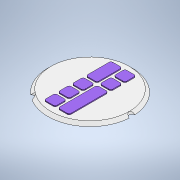
# Autodesk Inventor part: Лого ШП
Saved by Autodesk Inventor 2020 (Build 240168000, 168)
## iProperties
Created: 2021-06-18
Part Number: Лого ШП
Material: Типовые
Document SubType Name: Modeling
Designer: Антон
Density: 1 g/cm^3
Appearance: Белый
Author: Антон
Autodesk Inventor part; units mm, degrees
ref_plane "YZ Plane" through (0, 0, 0) normal (1, 0, 0) x (0, 1, 0)
ref_plane "XZ Plane" through (0, 0, 0) normal (0, 1, 0) x (-1, 0, 0)
ref_plane "XY Plane" through (0, 0, 0) normal (0, 0, 1) x (1, 0, 0)
sketch "Эскиз1" plane through (0, 0, 0) normal (0, 1, 0) x (-1, 0, 0)
  line L0 (0, 0) -> (23.1579, 0)
  line L1 (23.1579, 0) -> (23.1579, -40)
  line L2 (23.1579, -40) -> (0, -40)
  line L3 (0, -40) -> (0, 0)
  line L4 (17.9579, -3) -> (12.2807, -3)
  line L5 (12.2807, -3) -> (12.2807, -8.6772)
  line L6 (12.2807, -8.6772) -> (17.9579, -8.6772)
  line L7 (17.9579, -8.6772) -> (17.9579, -3)
  line L8 (17.9579, -10.0807) -> (12.2807, -10.0807)
  line L9 (12.2807, -10.0807) -> (12.2807, -15.7579)
  line L10 (12.2807, -15.7579) -> (17.9579, -15.7579)
  line L11 (17.9579, -15.7579) -> (17.9579, -10.0807)
  line L12 (17.9579, -17.1614) -> (12.2807, -17.1614)
  line L13 (12.2807, -17.1614) -> (12.2807, -22.8386)
  line L14 (12.2807, -22.8386) -> (17.9579, -22.8386)
  line L15 (17.9579, -22.8386) -> (17.9579, -17.1614)
  line L16 (17.9579, -24.2421) -> (12.2807, -24.2421)
  line L17 (12.2807, -24.2421) -> (12.2807, -37)
  line L18 (12.2807, -37) -> (17.9579, -37)
  line L19 (17.9579, -37) -> (17.9579, -24.2421)
  line L20 (10.8772, -24.2421) -> (5.2, -24.2421)
  line L21 (5.2, -24.2421) -> (5.2, -29.9193)
  line L22 (5.2, -29.9193) -> (10.8772, -29.9193)
  line L23 (10.8772, -29.9193) -> (10.8772, -24.2421)
  line L24 (10.8772, -31.3228) -> (5.2, -31.3228)
  line L25 (5.2, -31.3228) -> (5.2, -37)
  line L26 (5.2, -37) -> (10.8772, -37)
  line L27 (10.8772, -37) -> (10.8772, -31.3228)
  line L28 (10.8772, -3) -> (5.2, -3)
  line L29 (5.2, -3) -> (5.2, -22.8386)
  line L30 (5.2, -22.8386) -> (10.8772, -22.8386)
  line L31 (10.8772, -22.8386) -> (10.8772, -3)
  line L32 (15.1193, -8.6772) -> (15.1193, -10.0807)
  line L33 (15.1193, -15.7579) -> (15.1193, -17.1614)
  line L34 (15.1193, -22.8386) -> (15.1193, -24.2421)
  line L35 (8.0386, -22.8386) -> (8.0386, -24.2421)
  line L36 (8.0386, -29.9193) -> (8.0386, -31.3228)
  line L37 (15.1193, -3) -> (15.1193, 0)
  line L38 (15.1193, -37) -> (15.1193, -40)
  line L39 (17.9579, -12.9193) -> (23.1579, -12.9193)
  line L40 (5.2, -12.9193) -> (0, -12.9193)
  line L41 (12.2807, -12.9193) -> (10.8772, -12.9193)
  dimension "d0" = 23.1579
  dimension "d1" = 40
  dimension "d9" = 5.2
  dimension "d21" = 3
  constraints: 84 end point, 17 equal length, 16 midpoint, 16 parallel, 11 perpendicular, 9 collinear, 8 horizontal, 4 point on line, 1 vertical
  measures "d0" distance of L1.end L2.end
  measures "d1" distance of L0.end L1.end
  measures "d9" distance of L39.start L39.end
  measures "d21" distance of L37.start L37.end
extrude "Выдавливание1" add sketch "Эскиз1" along normal blind 0.5 contours L24 L27 L26 L25 | L20 L23 L22 L21 | L4 L7 L6 L5 | L29 L28 L31 L30 | L11 L10 L9 L8 | L18 L17 L16 L19 | L12 L15 L14 L13
sketch "Эскиз2" plane through (0, 0, 0) normal (0, -1, 0) x (1, 0, 0)
  line L0 (-5.2, -22.8386) -> (-10.8772, -22.8386) projected
  line L1 (-10.8772, -22.8386) -> (-10.8772, -3) projected
  line L2 (-10.8772, -3) -> (-5.2, -3) projected
  line L3 (-5.2, -3) -> (-5.2, -22.8386) projected
  line L4 (-5.2, -31.3228) -> (-5.2, -37) projected
  line L5 (-5.2, -37) -> (-10.8772, -37) projected
  line L6 (-10.8772, -37) -> (-10.8772, -31.3228) projected
  line L7 (-10.8772, -31.3228) -> (-5.2, -31.3228) projected
  line L8 (-17.9579, -17.1614) -> (-12.2807, -17.1614) projected
  line L9 (-12.2807, -22.8386) -> (-17.9579, -22.8386) projected
  line L10 (-17.9579, -22.8386) -> (-17.9579, -17.1614) projected
  line L11 (-17.9579, -37) -> (-17.9579, -24.2421) projected
  line L12 (-17.9579, -24.2421) -> (-12.2807, -24.2421) projected
  line L13 (-12.2807, -37) -> (-17.9579, -37) projected
  line L14 (-12.2807, -15.7579) -> (-17.9579, -15.7579) projected
  line L15 (-17.9579, -15.7579) -> (-17.9579, -10.0807) projected
  line L16 (-17.9579, -10.0807) -> (-12.2807, -10.0807) projected
  line L17 (-17.9579, -8.6772) -> (-17.9579, -3) projected
  line L18 (-17.9579, -3) -> (-12.2807, -3) projected
  line L19 (-12.2807, -8.6772) -> (-17.9579, -8.6772) projected
  line L20 (-5.2, -24.2421) -> (-5.2, -29.9193) projected
  line L21 (-5.2, -29.9193) -> (-10.8772, -29.9193) projected
  line L22 (-10.8772, -29.9193) -> (-10.8772, -24.2421) projected
  line L23 (-10.8772, -24.2421) -> (-5.2, -24.2421) projected
  line L24 (-12.2807, -17.1614) -> (-12.2807, -22.8386) projected
  line L25 (-12.2807, -24.2421) -> (-12.2807, -37) projected
  line L26 (-12.2807, -10.0807) -> (-12.2807, -15.7579) projected
  line L27 (-12.2807, -3) -> (-12.2807, -8.6772) projected
  line L28 (-10.8772, -3) -> (-5.2, -3) projected
  line L29 (-17.9579, -37) -> (-5.2, -3)
  circle A0 centre (-11.5789, -20) radius 21.35
  dimension "d24" = 42.7
  constraints: 2 end point, 1 centre point, 1 midpoint
  measures "d24" diameter of A0
extrude "Выдавливание2" add sketch "Эскиз2" along normal blind 1.5 contours L12 L25 L13 L29 | L29 L11 L12 | L24 L9 L29 | L29 L9 L10 L8 L24 | L0 L1 L29 L3 | L29 L1 L2 | L4 L5 L6 L7 | L14 L15 L16 L26 | L17 L18 L27 L19 | L20 L21 L22 L23 | A0
fillet "Сопряжение1" radius 1 28 edges at (-17.9579, 0.25, -3) (-17.9579, 0.25, -8.6772) (-12.2807, 0.25, -3) (-12.2807, 0.25, -8.6772) (-17.9579, 0.25, -15.7579) (-17.9579, 0.25, -10.0807) (-12.2807, 0.25, -10.0807) (-12.2807, 0.25, -15.7579) (-12.2807, 0.25, -22.8386) (-5.2, 0.25, -29.9193) (-5.2, 0.25, -22.8386) (-5.2, 0.25, -37) (-17.9579, 0.25, -22.8386) (-17.9579, 0.25, -37) (-10.8772, 0.25, -22.8386) (-10.8772, 0.25, -29.9193) (-10.8772, 0.25, -37) (-17.9579, 0.25, -24.2421) (-10.8772, 0.25, -3) (-12.2807, 0.25, -24.2421) (-5.2, 0.25, -24.2421) (-5.2, 0.25, -3) (-10.8772, 0.25, -24.2421) (-17.9579, 0.25, -17.1614) (-12.2807, 0.25, -17.1614) (-12.2807, 0.25, -37) (-10.8772, 0.25, -31.3228) (-5.2, 0.25, -31.3228)
chamfer "Фаска1" distance 1.5 angle 45 1 edges at (-32.9289, 0, -20)
sketch "Эскиз5" plane through (-11.5789, 0, -20) normal (0, 1, 0) x (1, 0, 0)
  circle A0 centre (0, 0) radius 19.85 projected
  circle A1 centre (0, 0) radius 21.35 projected
  circle A2 centre (21.35, 0) radius 1.5
  circle A3 centre (-12.7513, 17.1239) radius 1.5
  circle A4 centre (-12.7513, -17.1239) radius 1.5
  line L0 (28, 0) -> (-19.5959, 20)
  line L1 (28, 0) -> (-19.5959, -20)
  line L2 (-19.5959, 20) -> (-19.5959, -20)
  line L3 (0, 0) -> (-19.5959, 20)
  line L4 (0, 0) -> (-19.5959, -20)
  line L5 (28, 0) -> (0, 0)
  point P0 (11.5789, -20)
  dimension "d28" = 40
  dimension "d29" = 28
  constraints: 12 end point, 3 centre point, 3 equal length, 3 point on circle, 3 point on line, 3 tangent, 1 coincident, 1 horizontal
  measures "d28" distance of L0.end L1.end
  measures "d29" distance of L0.start A0.centre
extrude "Выдавливание5" cut sketch "Эскиз5" against normal blind 1.5 contours L5 A1 A2 | A2 A1 L5 | A2 L5 A1 | A1 L5 A2 | A3 A1 L0 | L0 A1 A3 | A1 L0 A3 | A4 L1 A1 | A4 A1 L1 | A4 L1 A1 | A3 L0 A1 | A1 L1 A4
equation "\"d0\" = 0.578947 * d1"
